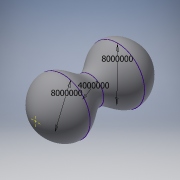
# Autodesk Inventor part: Haleys Comet
Saved by Autodesk Inventor 2017.2 (Build 212233000, 233)
## iProperties
Created: 2017-04-06
Part Number: Haleys Comet
Material: Water
Document SubType Name: Modeling
Designer: haden
Density: 0.9983 g/cm^3
Appearance: Default
Author: haden
Autodesk Inventor part; units mm, degrees
ref_plane "YZ Plane" through (0, 0, 0) normal (1, 0, 0) x (0, 1, 0)
sketch "Sketch1" plane through (0, 0, 0) normal (0, 0, 1) x (1, 0, 0)
  circle A0 centre (0, 0) radius 4000000
  dimension "d0" = 8000000
  constraints: 1 centre point, 1 coincident
  measures "d0" diameter of A0
ref_plane "Work Plane1" through (0, 0, 4000000) normal (0, 0, 1) x (1, 0, 0)
sketch "Sketch2" plane through (0, 0, 4000000) normal (0, 0, 1) x (1, 0, 0)
  circle A0 centre (0, 0) radius 2000000
  dimension "d2" = 4000000
  constraints: 1 centre point, 1 coincident
  measures "d2" diameter of A0
ref_plane "Work Plane2" through (0, 0, 8000000) normal (0, 0, 1) x (1, 0, 0)
sketch "Sketch3" plane through (0, 0, 8000000) normal (0, 0, 1) x (1, 0, 0)
  circle A0 centre (0, 0) radius 4000000
  dimension "d4" = 8000000
  constraints: 1 centre point, 1 coincident
  measures "d4" diameter of A0
ref_plane "Work Plane3" through (0, 0, 12000000) normal (0, 0, 1) x (1, 0, 0)
sketch "Sketch4" plane through (0, 0, 12000000) normal (0, 0, 1) x (1, 0, 0)
  point P0 (0, 0)
ref_plane "Work Plane4" through (0, 0, -4000000) normal (0, 0, 1) x (1, 0, 0)
sketch "Sketch5" plane through (0, 0, -4000000) normal (0, 0, 1) x (1, 0, 0)
  point P0 (0, 0)
sketch "Sketch6" plane through (0, 0, 0) normal (0, 1, 0) x (-1, 0, 0)
  line L0 (4000000, 8000000) -> (-4000000, 8000000) projected
  line L1 (2000000, 4000000) -> (-2000000, 4000000) projected
  line L2 (4000000, 0) -> (-4000000, 0) projected
  spline S0 degree 3 poles (0, 12000000) (-1885618.0832, 12000000) (-6100693.9017, 8145622.5515) (-189468.0252, 4000000) (-6100693.9017, -145622.5515) (-1885618.0832, -4000000) (0, -4000000) knots 0 0 0 0 565685.424949 1012899.020449 1460112.615949 2025798.040898 2025798.040898 2025798.040898 2025798.040898
  line L3 (0, 12000000) -> (100000, 12000000) construction
  line L4 (0, -4000000) -> (100000, -4000000) construction
  line L5 (0, 12000000) -> (0, -4000000)
  dimension "d10" = 100000
  dimension "d11" = 100000
  constraints: 6 end point, 4 horizontal, 1 vertical, 5 other
  measures "d10" distance of L3.start L3.end
  measures "d11" distance of L4.start L4.end
revolve "Revolution1" add sketch "Sketch6" angle 360 about axis through (0, 0, 12000000) along (0, 0, -1)
body "Solid1"
